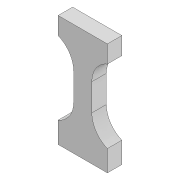
# Autodesk Inventor part: dogbone
Saved by Autodesk Inventor 2021 (Build 250183000, 183)
## iProperties
Created: 2021-07-02
Part Number: dogbone
Material: Generic
Document SubType Name: Modeling
Designer: mcgheealex
Density: 1 g/cm^3
Appearance: Default
Author: mcgheealex
Autodesk Inventor part; units mm, degrees
ref_plane "YZ Plane" through (0, 0, 0) normal (1, 0, 0) x (0, 1, 0)
ref_plane "XZ Plane" through (0, 0, 0) normal (0, 1, 0) x (-1, 0, 0)
ref_plane "XY Plane" through (0, 0, 0) normal (0, 0, 1) x (1, 0, 0)
sketch "Sketch1" plane through (0, 0, 0) normal (0, 0, 1) x (1, 0, 0)
  line L0 (-6.479, 14.2074) -> (6.479, 14.2074)
  line L1 (6.479, 14.2074) -> (6.479, -15.1712)
  line L2 (6.479, -15.1712) -> (-6.479, -15.1712)
  line L3 (-6.479, -15.1712) -> (-6.479, 14.2074)
  circle A0 centre (-8.9421, 3.5519) radius 6.5552
  circle A1 centre (8.9421, 3.5519) radius 6.5552
  line L4 (0, 0) -> (0, 6.0328) construction
  line L5 (-8.9421, 3.5519) -> (8.9421, 3.5519)
  line L6 (8.9421, 3.5519) -> (8.9421, -3.5519)
  line L7 (8.9421, -3.5519) -> (-8.9421, -3.5519)
  line L8 (-8.9421, -3.5519) -> (-8.9421, 3.5519)
  line L9 (0, 0) -> (1.9098, 0) construction
  circle A2 centre (8.9421, -3.5519) radius 6.5552
  circle A3 centre (-8.9421, -3.5519) radius 6.5552
  line L10 (-2.3869, 8.163) -> (2.3869, 8.163)
  line L11 (2.3869, 8.163) -> (2.3869, -7.3591)
  line L12 (2.3869, -7.3591) -> (-2.3869, -7.3591)
  line L13 (-2.3869, -7.3591) -> (-2.3869, 8.163)
  point P0 (-6.479, 9.6267)
  point P1 (-2.3869, 3.5519)
  point P2 (-2.3869, -3.5519)
  point P3 (-6.479, -9.6267)
  point P4 (6.479, -9.6267)
  point P5 (2.3869, -3.5519)
  point P6 (2.3869, 3.5519)
  point P7 (6.479, 9.6267)
  constraints: 28 end point, 6 parallel, 4 centre point, 4 horizontal, 4 tangent, 3 perpendicular, 2 coincident, 2 equal radius, 1 symmetric about line, 1 vertical, 2 other
extrude "Extrusion1" add sketch "Sketch1" along normal blind 3.81 contours L0 L1 A1 L11 L10 L13 A0 L3 | L13 L10 L11 L5 | L5 L11 L7 L13 | L13 L12 L11 A2 L1 L2 L3 A3 | L7 L11 L12 L13
body "Solid1"
